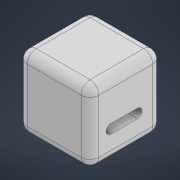
# Autodesk Inventor part: Head_prototype2
Saved by Autodesk Inventor 2021 (Build 250183000, 183)
## iProperties
Created: 2022-02-15
Part Number: Head_prototype2
Material: Generic
Document SubType Name: Modeling
Designer: utkaa
Density: 1 g/cm^3
Appearance: Default
Author: utkaa
Autodesk Inventor part; units mm, degrees
ref_plane "YZ Plane" through (0, 0, 0) normal (1, 0, 0) x (0, 1, 0)
ref_plane "XZ Plane" through (0, 0, 0) normal (0, 1, 0) x (-1, 0, 0)
ref_plane "XY Plane" through (0, 0, 0) normal (0, 0, 1) x (1, 0, 0)
sketch "Sketch1" plane through (0, 0, 0) normal (0, 0, 1) x (1, 0, 0)
  line L0 (100, 0) -> (700, 0)
  line L1 (800, -100) -> (800, -700)
  line L2 (700, -800) -> (100, -800)
  line L3 (0, -700) -> (0, -100)
  arc A0 (2, 0) -> (0, -2) centre (2, -2) ccw
  arc A1 (800, -100) -> (700, 0) centre (700, -100) ccw
  arc A2 (100, 0) -> (0, -100) centre (100, -100) ccw
  arc A3 (0, -700) -> (100, -800) centre (100, -700) ccw
  arc A4 (700, -800) -> (800, -700) centre (700, -700) ccw
  point P0 (0, 0)
  point P1 (800, -800)
  point P2 (0, -800)
  dimension "d0" = 800
  dimension "d1" = 800
  dimension "d2" = 2
  dimension "d3" = 100
  constraints: 10 point on circle, 10 tangent, 8 end point, 8 point on line, 5 centre point, 3 equal radius, 2 parallel, 1 horizontal, 1 perpendicular
  measures "d0" distance of point (800, -800) point (0, -800)
  measures "d1" distance between parallel lines of L2 L0
  measures "d2" radius of A0
  measures "d3" radius of A1
extrude "Extrusion1" add sketch "Sketch1" along normal blind 800
sketch "Sketch2" plane through (0, -700, 0) normal (-1, 0, 0) x (0, 0, 1)
  line L0 (250, 450) -> (550, 450)
  line L1 (550, 450) -> (550, 300)
  line L2 (550, 300) -> (250, 300)
  line L3 (250, 300) -> (250, 450)
  line L4 (0, 700) -> (800, 700) projected
  line L5 (0, -100) -> (800, -100) projected
  line L6 (800, 600) -> (800, 0) projected
  line L7 (0, 600) -> (0, 0) projected
  dimension "d6" = 300
  dimension "d7" = 150
  dimension "d8" = 250
  dimension "d9" = 400
  dimension "d10" = 250
  dimension "d11" = 250
  constraints: 8 end point, 2 parallel, 1 horizontal, 1 perpendicular
  measures "d6" distance of L1.end L2.end
  measures "d7" distance of L0.end L1.end
  measures "d8" distance between parallel lines of L0 L4
  measures "d9" distance between parallel lines of L5 L2
  measures "d10" distance between parallel lines of L6 L1
  measures "d11" distance between parallel lines of L7 L3
extrude "Extrusion2" cut sketch "Sketch2" against normal blind 200
fillet "Fillet1" radius 100 16 edges at (29.2893, -770.7107, 0) (400, -800, 0) (770.7107, -770.7107, 0) (800, -400, 0) (770.7107, -29.2893, 0) (400, 0, 0) (29.2893, -29.2893, 0) (0, -400, 0) (29.2893, -770.7107, 800) (400, -800, 800) (770.7107, -770.7107, 800) (800, -400, 800) (770.7107, -29.2893, 800) (400, 0, 800) (29.2893, -29.2893, 800) (0, -400, 800)
sketch "Sketch3" plane through (100, -800, 700) normal (0, -1, 0) x (1, 0, 0)
  circle A0 centre (300, -298.1465) radius 275
  line L0 (-100, -600) -> (-100, 0) projected
  line L1 (700, -600) -> (700, 0) projected
  point P0 (-100, -700)
  dimension "d15" = 550
  dimension "d16" = 400
  dimension "d17" = 400
  constraints: 1 centre point
  measures "d15" diameter of A0
  measures "d16" distance from line of L0 A0.centre
  measures "d17" distance from line of L1 A0.centre
extrude "Extrusion3" cut sketch "Sketch3" against normal blind 700
sketch "Sketch4" plane through (0, -700, 700) normal (-1, 0, 0) x (0, 0, 1)
  line L0 (-560.17, 235.0251) -> (-460.17, 235.0251)
  line L1 (-460.17, 235.0251) -> (-460.17, 205.0251)
  line L2 (-460.17, 205.0251) -> (-560.17, 205.0251)
  line L3 (-560.17, 205.0251) -> (-560.17, 235.0251)
  point P0 (-700, 700)
  dimension "d20" = 100
  dimension "d21" = 30
  constraints: 8 end point, 2 parallel, 1 horizontal, 1 perpendicular
  measures "d20" distance of L1.end L2.end
  measures "d21" distance of L0.end L1.end
extrude "Extrusion4" cut sketch "Sketch4" against normal blind 200
sketch "Sketch5" plane through (800, -700, 700) normal (1, 0, 0) x (0, 0, -1)
  line L0 (129.5986, 209.4371) -> (429.5986, 209.4371) construction
  line L1 (129.5986, 159.4371) -> (429.5986, 159.4371)
  line L2 (429.5986, 259.4371) -> (129.5986, 259.4371)
  arc A0 (129.5986, 259.4371) -> (129.5986, 159.4371) centre (129.5986, 209.4371) ccw
  arc A1 (429.5986, 159.4371) -> (429.5986, 259.4371) centre (429.5986, 209.4371) ccw
  point P0 (700, 700)
  point P1 (279.5986, 209.4371)
  dimension "d24" = 300
  dimension "d25" = 100
  constraints: 8 end point, 4 point on circle, 4 tangent, 2 centre point, 1 horizontal, 1 midpoint, 1 parallel
  measures "d24" distance of L0.start L0.end
  measures "d25" diameter of A1
extrude "Extrusion5" cut sketch "Sketch5" against normal blind 200
body "Solid1"
